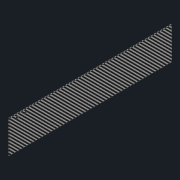
# Autodesk Inventor part: s_carbon_plate2
Saved by Autodesk Inventor 2021 (Build 250183000, 183)
## iProperties
Created: 2021-08-20
Part Number: s_carbon_plate2
Material: CFRP
Document SubType Name: Sheet Metal
Designer: yuta0
Density: 1.43 g/cm^3
Sheet Metal Rule: Default_mm
Appearance: カーボンファイバー
Author: yuta0
Autodesk Inventor part; units mm, degrees
ref_plane "YZ Plane" through (0, 0, 0) normal (1, 0, 0) x (0, 1, 0)
ref_plane "XZ Plane" through (0, 0, 0) normal (0, 1, 0) x (-1, 0, 0)
ref_plane "XY Plane" through (0, 0, 0) normal (0, 0, 1) x (1, 0, 0)
sketch "スケッチ1" plane through (0, 0, 0) normal (1, 0, 0) x (0, 1, 0)
  line L0 (-20, 100) -> (20, 100)
  line L1 (20, 100) -> (20, -100)
  line L2 (20, -100) -> (-20, -100)
  line L3 (-20, -100) -> (-20, 100)
  line L4 (-20, 100) -> (20, -100) construction
  line L5 (20, 100) -> (-20, -100) construction
  point P0 (0, 0)
  dimension "d0" = 40
  dimension "d1" = 200
  measures "d0" distance of L0.start L0.end
  measures "d1" distance of L0.end L1.end
extrude "プレート1" add sketch "スケッチ1" along normal mid plane 1
sketch "スケッチ2" plane through (0.5, 0, 0) normal (1, 0, 0) x (0, 0, -1)
  line L0 (-100, 20) -> (100, 20) projected
  line L1 (-100, -20) -> (-100, 20) projected
  point P0 (0, 0)
  point P1 (-90, 16)
  point P2 (-80, 16)
  dimension "d3" = 4
  dimension "d4" = 10
  dimension "d5" = 10
  constraints: 1 horizontal alignment
  measures "d3" distance from line of L0 point (-90, 16)
  measures "d4" distance from line of L1 point (-90, 16)
  measures "d5" distance of point (-90, 16) point (-80, 16)
hole "穴1" at (0.5, 16, 90) at (0.5, 16, 80) direction (-1, 0, 0) diameter 3.2 end through all clearance for "Socket Head Cap Screw" size "M3" standard "Ansi Metric M Profile"
equation "\"d11\" = Thickness"
equation "\"d2\" = Thickness"
equation "\"BendRadius\" = Thickness"
equation "\"BendReliefWidth\" = Thickness"
equation "\"BendReliefDepth\" = 0.5 * Thickness"
equation "\"CornerReliefSize\" = 4 * Thickness"
equation "\"MinimumRemnant\" = 2 * Thickness"
equation "\"TransitionRadius\" = BendRadius"
equation "\"JacobiRadiusSize\" = BendRadius"
equation "\"GapSize\" = Thickness"
equation "\"Thickness\" = 1"
